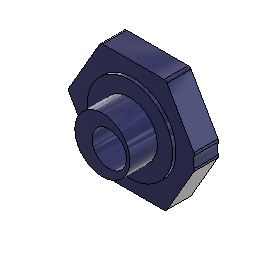
Excenter v1 (Autodesk Fusion 360 design; units mm, degrees)
Autodesk Fusion 360 part; units mm, degrees
sketch "Sketch1" plane through (0, 0, 0) normal (0, 0, 1) x (1, 0, 0)
  circle A0 centre (0, 0) radius 6.2
  circle A1 centre (0, 0) radius 4
  circle A2 centre (1, 0) radius 2.5
  line L0 (9.5, 0) -> (4.75, 8.2272)
  line L1 (4.75, 8.2272) -> (-4.75, 8.2272)
  line L2 (-4.75, 8.2272) -> (-9.5, 0)
  line L3 (-9.5, 0) -> (-4.75, -8.2272)
  line L4 (-4.75, -8.2272) -> (4.75, -8.2272)
  line L5 (4.75, -8.2272) -> (9.5, 0)
  line L6 (0, 0) -> (1, 0) construction
  circle A3 centre (11.7511, 0) radius 3
  line L7 (9.5, 0) -> (11.7511, 0) construction
  line L8 (8.9226, 1) -> (8.9226, -1) construction
  dimension "d1" = 16.4545
  dimension "d2" = 12.4
  dimension "d3" = 8
  dimension "d4" = 5
  dimension "d5" = 1
  dimension "d6" = 6
  dimension "d7" = 2
  measures "d1" distance of L1 L4
  measures "d2" diameter of A0
  measures "d3" diameter of A1
  measures "d4" diameter of A2
  measures "d5" distance of A0.centre A2.centre
  measures "d6" diameter of A3
  measures "d7" distance of L8.start L8.end
extrude "Extrude1" add sketch "Sketch1" along normal blind 8 contours A1
extrude "Extrude2" add sketch "Sketch1" along normal blind 3.5 contours A0 | L0 L1 L2 L3 L4 L5 A3
extrude "Extrude3" add sketch "Sketch1" along normal blind 0.5 from surface at 3.5 contours A0
fillet "Fillet1" radius 0.5 5 edges at (4.75, -8.2272, 1.75) (-4.75, -8.2272, 1.75) (-9.5, 0, 1.75) (-4.75, 8.2272, 1.75) (4.75, 8.2272, 1.75)
fillet "Fillet2" radius 0.5 2 edges at (8.9226, 1, 1.75) (8.9226, -1, 1.75)
sketch "Sketch2" plane through (0, 0, 0) normal (0, 0, 1) x (1, 0, 0)
  circle A0 centre (1, 0) radius 2.5
  arc A1 (8.8128, -1.1903) -> (8.8614, -0.806) centre (8.3798, -0.9403) ccw
  line L0 (8.8128, -1.1903) -> (4.8943, -7.9772)
  arc A2 (4.4613, -8.2272) -> (4.8943, -7.9772) centre (4.4613, -7.7272) ccw
  line L1 (4.4613, -8.2272) -> (-4.4613, -8.2272)
  arc A3 (-4.8943, -7.9772) -> (-4.4613, -8.2272) centre (-4.4613, -7.7272) ccw
  line L2 (-4.8943, -7.9772) -> (-9.3557, -0.25)
  arc A4 (-9.3557, 0.25) -> (-9.3557, -0.25) centre (-8.9226, 0) ccw
  line L3 (-9.3557, 0.25) -> (-4.8943, 7.9772)
  arc A5 (-4.4613, 8.2272) -> (-4.8943, 7.9772) centre (-4.4613, 7.7272) ccw
  line L4 (-4.4613, 8.2272) -> (4.4613, 8.2272)
  arc A6 (4.8943, 7.9772) -> (4.4613, 8.2272) centre (4.4613, 7.7272) ccw
  line L5 (4.8943, 7.9772) -> (8.8128, 1.1903)
  arc A7 (8.8614, 0.806) -> (8.8128, 1.1903) centre (8.3798, 0.9403) ccw
  arc A8 (8.8614, 0.806) -> (8.8614, -0.806) centre (11.7511, 0) ccw
  circle A9 centre (0, 0) radius 4
  circle A10 centre (0, 0) radius 6.2
